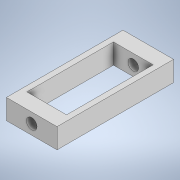
# Autodesk Inventor part: MM3_cage
Saved by Autodesk Inventor 2021 (Build 250183000, 183)
## iProperties
Created: 2021-02-23
Part Number: MM3_cage
Material: Generic
Document SubType Name: Modeling
Designer: dsdan
Density: 1 g/cm^3
Appearance: Default
Author: dsdan
Autodesk Inventor part; units mm, degrees
ref_plane "YZ Plane" through (0, 0, 0) normal (1, 0, 0) x (0, 1, 0)
ref_plane "XZ Plane" through (0, 0, 0) normal (0, 1, 0) x (-1, 0, 0)
ref_plane "XY Plane" through (0, 0, 0) normal (0, 0, 1) x (1, 0, 0)
sketch "Sketch1" plane through (0, 0, 0) normal (0, 1, 0) x (-1, 0, 0)
  line L0 (9.55, 22) -> (-9.55, 22)
  line L1 (-9.55, 22) -> (-9.55, -22)
  line L2 (-9.55, -22) -> (9.55, -22)
  line L3 (9.55, -22) -> (9.55, 22)
  line L4 (9.55, 22) -> (-9.55, -22) construction
  line L5 (-9.55, 22) -> (9.55, -22) construction
  line L6 (7.5, 16.35) -> (-7.5, 16.35)
  line L7 (-7.5, 16.35) -> (-7.5, -16.35)
  line L8 (-7.5, -16.35) -> (7.5, -16.35)
  line L9 (7.5, -16.35) -> (7.5, 16.35)
  line L10 (7.5, 16.35) -> (-7.5, -16.35) construction
  line L11 (-7.5, 16.35) -> (7.5, -16.35) construction
  point P0 (0, 0)
  dimension "d0" = 44
  dimension "d1" = 19.1
  dimension "d4" = 32.7
  dimension "d5" = 15
  constraints: 24 end point, 4 midpoint, 4 parallel, 2 horizontal, 2 perpendicular
  measures "d0" distance of L1.end L0.end
  measures "d1" distance of L1.end L2.end
  measures "d4" distance of L7.end L6.end
  measures "d5" distance between parallel lines of L7 L9
extrude "Extrusion1" add sketch "Sketch1" along normal blind 7.6
sketch "Sketch2" plane through (-9.55, 0, 22) normal (0, 0, 1) x (1, 0, 0)
  circle A0 centre (9.55, 3.8) radius 2
  line L0 (0, 0) -> (0, 7.6) projected
  line L1 (0, 7.6) -> (19.1, 0) construction
  line L2 (19.1, 0) -> (0, 0) projected
  line L3 (19.1, 7.6) -> (0, 0) construction
  point P0 (9.55, 0)
  dimension "d6" = 4
  constraints: 4 end point, 1 centre point, 1 midpoint
  measures "d6" diameter of A0
extrude "Extrusion2" cut sketch "Sketch2" against normal through all
body "Solid1"
